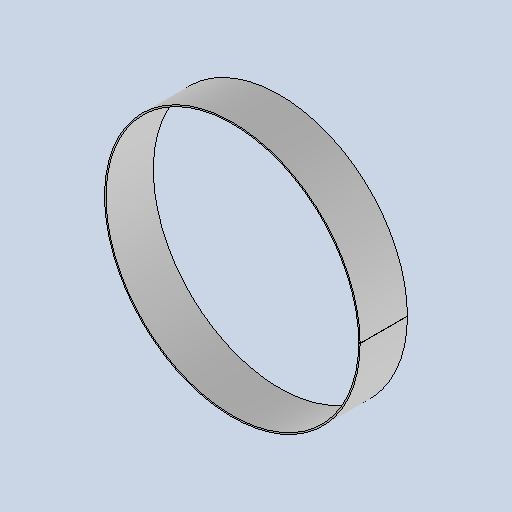
# Autodesk Inventor part: MSC 402 RING
Saved by Autodesk Inventor 2025 (Build 290162010, 162A)
## iProperties
Created: 2024-06-19
Part Number: MSC 402 RING
Material: Stainless Steel
Document SubType Name: Sheet Metal
Designer: pokla
Density: 8 g/cm^3
Flat Pattern Width: 168.544 cm
Flat Pattern Length: 10 cm
Flat Pattern Area: 1685.44 cm^2
Sheet Metal Rule: AISI304 3mm Die 32
Sheet Metal Width: 1685,436 mm
Sheet Metal Length: 100,000 mm
Sheet Metal Area: 168543,597 mm^2
Appearance: Default
Stock Number: МОО 402 кольцо
Mass: 4047.76 g
Surface Area: 3480.33 cm^2
Volume: 505.97 cm^3
Author: pokla
Autodesk Inventor part; units mm, degrees
ref_plane "YZ Plane" through (0, 0, 0) normal (1, 0, 0) x (0, 1, 0)
ref_plane "XZ Plane" through (0, 0, 0) normal (0, 1, 0) x (-1, 0, 0)
ref_plane "XY Plane" through (0, 0, 0) normal (0, 0, 1) x (1, 0, 0)
sketch "Sketch3" plane through (0, 0, 0) normal (0, 0, 1) x (1, 0, 0)
  line L0 (-270, 50) -> (-267, 50)
  line L1 (-267, 50) -> (-267, -50)
  line L2 (-267, -50) -> (-270, -50)
  line L3 (-270, -50) -> (-270, 50)
  line L4 (0, -70) -> (0, 70) projected
  point P0 (0, 0)
  point P1 (-270, 0)
  dimension "d1" = 3
  dimension "d2" = 100
  dimension "d3" = 270
  constraints: 8 end point, 2 parallel, 1 horizontal, 1 horizontal alignment, 1 midpoint, 1 perpendicular
  measures "d1" distance of L0.start L0.end
  measures "d2" distance of L2.end L0.start
  measures "d3" distance of point (0, 0) point (-270, 0)
revolve "Revolution1" add sketch "Sketch3" angle 359.9 mid plane about axis through (0, -10, 0) along (0, 1, 0)
equation "\"BendReliefWidth\" = Thickness"
equation "\"BendReliefDepth\" = 0.5 * Thickness"
equation "\"CornerReliefSize\" = 4 * Thickness"
equation "\"MinimumRemnant\" = 2 * Thickness"
equation "\"TransitionRadius\" = BendRadius"
equation "\"JacobiRadiusSize\" = BendRadius"
equation "\"GapSize\" = Thickness"
equation "\"Thickness\" = 3"
equation "\"BendRadius\" = 5"
body "Solid1"
